Tapeziertisch halter (Autodesk Fusion 360 design; units mm, degrees)
Autodesk Fusion 360 part; units mm, degrees
sketch "Sketch1" plane through (0, 0, 0) normal (0, 0, 1) x (1, 0, 0)
  line L0 (0, 0) -> (160, 0)
  circle A0 centre (0, 0) radius 3
  circle A1 centre (160, 0) radius 3
  circle A2 centre (0, 0) radius 9
  circle A3 centre (160, 0) radius 9
  line L1 (-9, 9) -> (169, 9)
  line L2 (169, 9) -> (169, -9)
  line L3 (169, -9) -> (-9, -9)
  line L4 (-9, -9) -> (-9, 9)
  line L5 (-3, 9) -> (3, 9)
  line L6 (3, 9) -> (3, -3)
  line L7 (3, -3) -> (-3, -3)
  line L8 (-3, -3) -> (-3, 9)
  line L9 (157, 3) -> (163, 3)
  line L10 (163, 3) -> (163, -9)
  line L11 (163, -9) -> (157, -9)
  line L12 (157, -9) -> (157, 3)
  dimension "d1" = 160
  dimension "d2" = 6
  dimension "d3" = 6
  dimension "d4" = 18
  dimension "d5" = 18
  constraint coincident L0.start A0.centre
  constraint horizontal L0
  constraint coincident L0.end A1.centre
  constraint concentric A0 A2
  constraint concentric A1 A3
  constraint horizontal L1
  constraint vertical L2
  constraint horizontal L3
  constraint vertical L4
  constraint tangent A2 L4
  constraint tangent A2 L1
  constraint tangent A3 L2
  constraint tangent A3 L3
  constraint horizontal L5
  constraint vertical L6
  constraint horizontal L7
  constraint vertical L8
  constraint tangent A0 L7
  constraint tangent A2 L5
  constraint tangent A0 L6
  constraint tangent A0 L8
  constraint horizontal L9
  constraint vertical L10
  constraint horizontal L11
  constraint vertical L12
  constraint tangent A1 L9
  constraint tangent A1 L12
  constraint tangent A1 L10
  constraint tangent A3 L11
  measures "d1" distance of L0.start L0.end
  measures "d2" diameter of A0
  measures "d3" diameter of A1
  measures "d4" diameter of A2
  measures "d5" diameter of A3
extrude "Extrude1" add sketch "Sketch1" along normal blind 4 contours L0 A2 L6 | A0 L6 L7 | L0 A2 L6 L7 L8 | L0 A2 A3 L1 L6 | L0 A2 A3 L3 L12 | A0 L7 L8 | L0 A3 L9 L10 L12 | L0 A3 L12 | A2 L1 L4 L8 | A1 L9 L12 | A1 L9 L10 | A3 L2 L3 L10
fillet "Fillet1" radius 5 2 edges at (157, -9, 2) (3, 9, 2)
